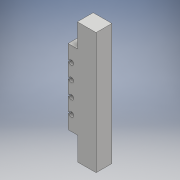
# Autodesk Inventor part: PiezaInferior
Saved by Autodesk Inventor 2017 (Build 210142000, 142)
## iProperties
Created: 2021-02-12
Part Number: PiezaInferior
Material: Generic
Document SubType Name: Modeling
Designer: USUARIO
Density: 1 g/cm^3
Appearance: Default
Author: USUARIO
Autodesk Inventor part; units mm, degrees
ref_plane "YZ Plane" through (0, 0, 0) normal (1, 0, 0) x (0, 1, 0)
ref_plane "XZ Plane" through (0, 0, 0) normal (0, 1, 0) x (-1, 0, 0)
ref_plane "XY Plane" through (0, 0, 0) normal (0, 0, 1) x (1, 0, 0)
sketch "Sketch3" plane through (0, 0, 0) normal (0, 1, 0) x (-1, 0, 0)
  line L0 (0, -389.8459) -> (0, 0)
  line L1 (60.3256, -0.2092) -> (60.0656, -75.2087)
  line L2 (60.0656, -75.2087) -> (90.0654, -75.3128)
  line L3 (58.9739, -390.0504) -> (59.2339, -315.0509)
  line L4 (59.2339, -315.0509) -> (89.2337, -315.1549)
  line L5 (0, 0) -> (60.3256, -0.2092)
  line L6 (60.0656, -75.2087) -> (90.0654, -75.3128)
  line L7 (60.0656, -75.2087) -> (60.3256, -0.2092)
  line L8 (90.0654, -75.3128) -> (89.2337, -315.1549)
  line L9 (59.2339, -315.0509) -> (89.2337, -315.1549)
  line L10 (59.2339, -315.0509) -> (58.9739, -390.0504)
  line L11 (58.9739, -390.0504) -> (0, -389.8459)
  circle A0 centre (79.899, -123.2778) radius 7.5
  circle A1 centre (79.7326, -171.2775) radius 7.5
  circle A2 centre (79.5661, -219.2772) radius 7.5
  circle A3 centre (79.3997, -267.2769) radius 7.5
  line L12 (89.9043, -121.7778) -> (86.9043, -121.7778)
  line L13 (86.9043, -121.7778) -> (86.9043, -124.7778)
  line L14 (86.9043, -124.7778) -> (89.9043, -124.7778)
  line L15 (89.9043, -124.7778) -> (89.9043, -121.7778)
  line L16 (86.7378, -169.7775) -> (86.7378, -172.7775)
  line L17 (89.7378, -169.7775) -> (86.7378, -169.7775)
  line L18 (86.7378, -172.7775) -> (89.7378, -172.7775)
  line L19 (89.7378, -172.7775) -> (89.7378, -169.7775)
  line L20 (86.5714, -217.7772) -> (86.5714, -220.7772)
  line L21 (89.5714, -217.7772) -> (86.5714, -217.7772)
  line L22 (86.5714, -220.7772) -> (89.5714, -220.7772)
  line L23 (89.5714, -220.7772) -> (89.5714, -217.7772)
  line L24 (86.405, -265.7769) -> (86.405, -268.7769)
  line L25 (89.405, -265.7769) -> (86.405, -265.7769)
  line L26 (86.405, -268.7769) -> (89.405, -268.7769)
  line L27 (89.405, -268.7769) -> (89.405, -265.7769)
  dimension "d2" = 30
  dimension "d3" = 75
  dimension "d4" = 30
  dimension "d5" = 75
  dimension "d6" = 15
  dimension "d12" = 48
  dimension "d14" = 48
  dimension "d15" = 10
  dimension "d16" = 3
  dimension "d17" = 3
  dimension "d18" = 1.5
  dimension "d24" = 48
  constraints: 56 end point, 4 centre point, 3 collinear, 3 parallel, 3 perpendicular, 1 horizontal, 1 point on line, 32 other
  measures "d2" distance of L2.end L1.end
  measures "d3" distance of L1.end L1.start
  measures "d4" distance of L3.end L4.end
  measures "d5" distance of L3.start L3.end
  measures "d6" diameter of A0
  measures "d12" distance of A0.centre A1.centre
  measures "d14" distance from line of L2 A0.centre
  measures "d15" distance from line of L8 A0.centre
  measures "d16" distance of L14.end L13.end
  measures "d17" distance of L13.end L12.end
  measures "d18" distance from line of L12 A0.centre
  measures "d24" distance of L12.end L16.start
extrude "Extrusion1" add sketch "Sketch3" along normal blind 50.8 contours L0 L5 L1 L2 L8 L12 A0 L14 L17 A1 L18 L21 A2 L22 L25 A3 L26 L4 L3 L11 | L26 A3 L25 L8 | L8 L14 A0 L12 | L22 A2 L21 L8 | L8 L18 A1 L17
sketch "Sketch4" plane through (0, 50.8, 0) normal (0, 1, 0) x (1, 0, 0)
  line L0 (-89.2337, 315.1549) -> (-90.0654, 75.3128) projected
  line L1 (-89.9077, 120.7778) -> (-86.9077, 120.7778)
  line L2 (-86.9077, 120.7778) -> (-86.9077, 125.7778)
  line L3 (-86.9077, 125.7778) -> (-89.9077, 125.7778)
  line L4 (-89.9077, 125.7778) -> (-89.9077, 120.7778)
  line L5 (-86.7413, 168.7775) -> (-86.7413, 173.7775)
  line L6 (-86.7413, 173.7775) -> (-89.7413, 173.7775)
  line L7 (-89.7413, 168.7775) -> (-86.7413, 168.7775)
  line L8 (-89.7413, 173.7775) -> (-89.7413, 168.7775)
  line L9 (-86.5749, 216.7772) -> (-86.5749, 221.7772)
  line L10 (-86.5749, 221.7772) -> (-89.5749, 221.7772)
  line L11 (-89.5749, 216.7772) -> (-86.5749, 216.7772)
  line L12 (-89.5749, 221.7772) -> (-89.5749, 216.7772)
  line L13 (-86.4084, 264.7769) -> (-86.4084, 269.7769)
  line L14 (-86.4084, 269.7769) -> (-89.4084, 269.7769)
  line L15 (-89.4084, 264.7769) -> (-86.4084, 264.7769)
  line L16 (-89.4084, 269.7769) -> (-89.4084, 264.7769)
  circle A0 centre (-79.899, 123.2778) radius 7.5 projected
  point P0 (0, 0)
  dimension "d28" = 3
  dimension "d29" = 5
  dimension "d35" = 48
  dimension "d39" = 2.5
  constraints: 32 end point, 2 parallel, 1 horizontal, 1 perpendicular, 1 point on line, 25 other
  measures "d28" distance of L3.end L2.end
  measures "d29" distance of L2.end L1.end
  measures "d35" distance of L1.end L5.start
  measures "d39" distance from line of A0.centre L1
extrude "Extrusion2" cut sketch "Sketch4" against normal blind 50.8 contours L14 L13 L15 L0 | L0 L16 L14 | L10 L9 L11 L0 | L0 L12 L10 | L6 L5 L7 L0 | L0 L8 L6 | L3 A0 L1 L0 | L0 L4 L3 | L3 L2 L1 A0 picked at (-87.0554, 123.5604)
body "Solid1"
